Autodesk Inventor part; units mm, degrees
(part 2 of 2)
  line L848 (1018.2668, 182.8734) -> (1018.5668, 182.9484)
  line L849 (1018.5668, 182.9484) -> (1018.8668, 183.0734)
  line L850 (1018.8668, 183.0734) -> (1019.1668, 183.1985)
  line L851 (1019.1668, 183.1985) -> (1019.4668, 183.3485)
  line L852 (1019.4668, 183.3485) -> (1019.7418, 183.5235)
  line L853 (1019.7418, 183.5235) -> (1020.0167, 183.7236)
  line L854 (1020.0167, 183.7236) -> (1020.2666, 183.9237)
  line L855 (1020.2666, 183.9237) -> (1020.4917, 184.1486)
  line L856 (1020.4917, 184.1486) -> (1020.7167, 184.3986)
  line L857 (1020.7167, 184.3986) -> (1020.9168, 184.6485)
  line L858 (1020.9168, 184.6485) -> (1021.1168, 184.9235)
  line L859 (1021.1168, 184.9235) -> (1021.2919, 185.1985)
  line L860 (1021.2919, 185.1985) -> (1021.442, 185.4734)
  line L861 (1021.442, 185.4734) -> (1021.5921, 185.7733)
  line L862 (1021.5921, 185.7733) -> (1021.6922, 186.0733)
  line L863 (1021.6922, 186.0733) -> (1021.7924, 186.3983)
  line L864 (1021.7924, 186.3983) -> (1021.8674, 186.7233)
  line L865 (1021.8674, 186.7233) -> (1021.9176, 187.0482)
  line L866 (1021.9176, 187.0482) -> (1021.9427, 187.3732)
  line L867 (1021.9427, 187.3732) -> (1021.9678, 187.6982)
  line L868 (1021.9678, 187.6982) -> (1021.9678, 237.6982)
  line L869 (1021.9678, 237.6982) -> (1021.9429, 238.0232)
  point P0 (0, 0)
  constraints: 1692 end point, 476 parallel, 195 perpendicular, 8 collinear, 1 horizontal, 21 other
extrude "Extrusion1" add sketch "Sketch1" along normal blind 6 contours L81 L80 L79 L78 L77 L76 L75 L74 L73 L72 L71 L70 L69 L68 L67 L66 L65 L64 L63 L62 L61 L60 L59 L58 L57 L56 L55 L54 L53 L52 L51 L50 L49 L48 L47 L46 L45 S6 S5 S4 S3 S2 S1 S0 L20 L19 L18 L17 L16 L15 L14 L13 L12 L11 L10 L9 L8 L7 L6 L5 L4 L3 L2 L1 L0
body "Solid1"
